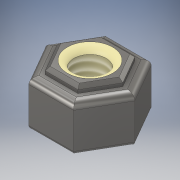
# Autodesk Inventor part: 10-24_Nut
Saved by Autodesk Inventor 2019 (Build 230136000, 136)
## iProperties
Created: 2021-01-31
Part Number: 10-24_Nut
Material: Steel, Alloy
Document SubType Name: Modeling
Designer: zhanb
Density: 7.73 g/cm^3
Appearance: Semi-Polished
Author: zhanb
Autodesk Inventor part; units mm, degrees
ref_plane "YZ Plane" through (0, 0, 0) normal (1, 0, 0) x (0, 1, 0)
ref_plane "XZ Plane" through (0, 0, 0) normal (0, 1, 0) x (-1, 0, 0)
ref_plane "XY Plane" through (0, 0, 0) normal (0, 0, 1) x (1, 0, 0)
sketch "Sketch1" plane through (0, 0, 0) normal (0, 1, 0) x (-1, 0, 0)
  line L0 (-2.7496, -4.7625) -> (-5.4993, 0)
  line L1 (-5.4993, 0) -> (-2.7496, 4.7625)
  line L2 (-2.7496, 4.7625) -> (2.7496, 4.7625)
  line L3 (2.7496, 4.7625) -> (5.4993, 0)
  line L4 (5.4993, 0) -> (2.7496, -4.7625)
  line L5 (2.7496, -4.7625) -> (-2.7496, -4.7625)
  point P0 (0, 0)
  point P1 (0, 0)
  dimension "d0" = 9.525
  constraints: 12 end point, 1 coincident, 1 horizontal, 13 other
  measures "d0" distance between parallel lines of L2 L5
extrude "Extrusion1" add sketch "Sketch1" along normal blind 6.35
sketch "Sketch2" plane through (0, 6.35, 0) normal (0, 1, 0) x (1, 0, 0)
  line L0 (5.4993, 0) -> (2.7496, 4.7625) projected
  line L1 (2.7496, 4.7625) -> (-2.7496, 4.7625) projected
  line L2 (-2.7496, 4.7625) -> (-5.4993, 0) projected
  line L3 (-5.4993, 0) -> (-2.7496, -4.7625) projected
  line L4 (-2.7496, -4.7625) -> (2.7496, -4.7625) projected
  line L5 (2.7496, -4.7625) -> (5.4993, 0) projected
  line L6 (-4.0328, 0) -> (-2.0164, 3.4925)
  line L7 (-2.0164, 3.4925) -> (2.0164, 3.4925)
  line L8 (2.0164, 3.4925) -> (4.0328, 0)
  line L9 (4.0328, 0) -> (2.0164, -3.4925)
  line L10 (2.0164, -3.4925) -> (-2.0164, -3.4925)
  line L11 (-2.0164, -3.4925) -> (-4.0328, 0)
  point P0 (0, 0)
  point P1 (0, 0)
  dimension "d3" = 1.27
  constraints: 12 end point, 1 coincident, 1 horizontal, 13 other
  measures "d3" distance between parallel lines of L4 L10
extrude "Extrusion2" cut sketch "Sketch2" against normal blind 0.7937
fillet "Fillet1" radius 0.7937 6 edges at (0, 5.5562, 4.7625) (4.1244, 5.5562, -2.3812) (0, 5.5562, -4.7625) (-4.1244, 5.5562, -2.3813) (-4.1244, 5.5562, 2.3812) (4.1244, 5.5562, 2.3813)
chamfer "Chamfer1" distance 0.3969 angle 45 6 edges at (3.0246, 6.35, 1.7463) (0, 6.35, 3.4925) (-3.0246, 6.35, 1.7463) (-3.0246, 6.35, -1.7462) (0, 6.35, -3.4925) (3.0246, 6.35, -1.7463)
sketch "Sketch3" plane through (0, 6.35, 0) normal (0, 1, 0) x (1, 0, 0)
  point P0 (0, 0)
  point P1 (0, 0)
  constraints: 1 coincident
hole "Hole1" at (0, 6.35, 0) direction (0, -1, 0) diameter 3.9688 end through all
fillet "Fillet2" radius 0.7937 1 edges at (0, 6.35, -1.9844)
thread "Thread1" size "10-24 UNC" class "2B" standard "ANSI Unified Screw Threads" full length
chamfer "Chamfer2" distance 0.3969 angle 45 1 edges at (0, 0, -1.9844)
fillet "Fillet3" radius 0.3969 6 edges at (4.1244, 0, 2.3813) (4.1244, 0, -2.3812) (0, 0, 4.7625) (-4.1244, 0, 2.3812) (-4.1244, 0, -2.3813) (0, 0, -4.7625)
body "Solid1"
